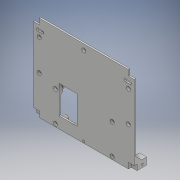
# Autodesk Inventor part: baseplate_jetson_core
Saved by Autodesk Inventor 2018 (Build 220112000, 112)
## iProperties
Created: 2018-05-14
Part Number: baseplate_jetson_core
Material: Generic
Document SubType Name: Modeling
Designer: bitbots
Density: 1 g/cm^3
Appearance: Default
Author: bitbots
Autodesk Inventor part; units mm, degrees
ref_plane "YZ Plane" through (0, 0, 0) normal (1, 0, 0) x (0, 1, 0)
ref_plane "XZ Plane" through (0, 0, 0) normal (0, 1, 0) x (-1, 0, 0)
ref_plane "XY Plane" through (0, 0, 0) normal (0, 0, 1) x (1, 0, 0)
sketch "Sketch1" plane through (0, 0, 0) normal (0, 1, 0) x (-1, 0, 0)
  line L0 (-70, 60) -> (70, 60)
  line L1 (70, 60) -> (70, -60)
  line L2 (70, -60) -> (-70, -60)
  line L3 (-70, -60) -> (-70, 60)
  line L4 (-70, 60) -> (70, -60) construction
  line L5 (70, 60) -> (-70, -60) construction
  point P0 (0, 0)
  dimension "d0" = 140
  dimension "d1" = 120
  constraints: 12 end point, 2 midpoint, 2 parallel, 1 horizontal, 1 perpendicular
  measures "d0" distance of L1.end L2.end
  measures "d1" distance of L0.end L1.end
extrude "Extrusion1" add sketch "Sketch1" along normal blind 2
sketch "Sketch2" plane through (0, 2, 0) normal (0, 1, 0) x (1, 0, 0)
  line L0 (0, 0) -> (0, 14) construction
  line L1 (0, 14) -> (39.5, 14) construction
  line L2 (39.5, 14) -> (-39.5, 14) construction
  line L3 (-39.5, 14) -> (-39.5, 56) construction
  line L4 (-39.5, 56) -> (39.5, 56) construction
  line L5 (39.5, 56) -> (39.5, 14) construction
  circle A0 centre (-39.5, 56) radius 1.75
  circle A1 centre (-39.5, 14) radius 1.75
  circle A2 centre (39.5, 14) radius 1.75
  circle A3 centre (39.5, 56) radius 1.75
  line L6 (70, 60) -> (-70, 60) projected
  dimension "d5" = 39.5
  dimension "d6" = 79
  dimension "d7" = 42
  dimension "d8" = 3.5
  dimension "d9" = 3.5
  dimension "d10" = 3.5
  dimension "d11" = 3.5
  dimension "d36" = 4
  constraints: 12 end point, 4 centre point, 4 coincident, 2 parallel, 2 perpendicular, 1 horizontal, 1 vertical
  measures "d5" distance of L0.end L1.end
  measures "d6" distance of L3.end L4.end
  measures "d7" distance of L2.end L3.end
  measures "d8" diameter of A0
  measures "d9" diameter of A1
  measures "d10" diameter of A2
  measures "d11" diameter of A3
  measures "d36" distance between parallel lines of L6 L4
extrude "Extrusion2" cut sketch "Sketch2" against normal through all
sketch "Sketch6" plane through (0, 2, 0) normal (0, 1, 0) x (1, 0, 0)
  circle A0 centre (39.5, 14) radius 1.75 projected
  circle A1 centre (-39.5, 56) radius 1.75 projected
  circle A2 centre (-39.5, 14) radius 1.75 projected
  circle A3 centre (39.5, 56) radius 1.75 projected
  line L0 (-70, -60) -> (70, -60) projected
  line L1 (70, -60) -> (70, 60) projected
  line L2 (70, 60) -> (-70, 60) projected
  line L3 (-70, 60) -> (-70, -60) projected
  line L4 (70, 60) -> (70, -60) projected
  line L5 (70, 60) -> (60, 60)
  line L6 (60, 60) -> (60, 50)
  line L7 (60, 50) -> (70, 50)
  line L8 (70, 50) -> (70, 60)
  point P0 (0, 0)
  dimension "d49" = 10
  dimension "d50" = 10
  constraints: 8 end point, 2 parallel, 1 horizontal, 1 perpendicular
  measures "d49" distance of L7.end L6.end
  measures "d50" distance of L6.end L5.end
extrude "Extrusion6" add sketch "Sketch6" along normal blind 15 contours L7 L6 L2 L1
sketch "Sketch8" plane through (70, 0, 60) normal (1, 0, 0) x (0, 0, -1)
  line L0 (120, 0) -> (0, 0) projected
  line L1 (120, 0) -> (120, 17) projected
  line L2 (110, 17) -> (120, 17) projected
  line L3 (110, 2) -> (110, 17) projected
  line L4 (0, 2) -> (110, 2) projected
  line L5 (0, 0) -> (0, 2) projected
  line L6 (110, 2) -> (110, 11)
  line L7 (110, 2) -> (110, 17) projected
  line L8 (110, 11) -> (116, 11)
  circle A0 centre (116, 11) radius 1.5
  point P0 (60, 0)
  dimension "d56" = 9
  dimension "d57" = 6
  dimension "d58" = 3
  constraints: 4 end point, 1 centre point, 1 coincident, 1 perpendicular, 1 point on line
  measures "d56" distance of L3.start L6.end
  measures "d57" distance of L6.end L8.end
  measures "d58" diameter of A0
extrude "Extrusion8" cut sketch "Sketch8" against normal blind 10 contours A0
mirror "Mirror1" about plane through (0, 0, 0) normal (1, 0, 0) of "Extrusion6", "Extrusion8"
chamfer "Chamfer1" distance 8 angle 45 4 edges at (-60, 2, -55) (60, 2, -55) (-65, 2, -50) (65, 2, -50)
sketch "Sketch9" plane through (0, 0, 0) normal (0, -1, 0) x (1, 0, 0)
  circle A0 centre (39.5, -14) radius 1.75 projected
  circle A1 centre (-39.5, -56) radius 1.75 projected
  circle A2 centre (-39.5, -14) radius 1.75 projected
  circle A3 centre (39.5, -56) radius 1.75 projected
  line L0 (70, 60) -> (-70, 60) projected
  line L1 (-70, 60) -> (-70, -60) projected
  line L2 (-70, -60) -> (70, -60) projected
  line L3 (70, -60) -> (70, 60) projected
  line L4 (-70, 60) -> (-70, -60) projected
  line L5 (-70, -60) -> (-62, -60)
  line L6 (-62, -60) -> (-62, -52)
  line L7 (-62, -52) -> (-70, -52)
  line L8 (-70, -52) -> (-70, -60)
  line L9 (70, -60) -> (60, -60) projected
  line L10 (70, -60) -> (60, -60)
  line L11 (70, -50) -> (70, -60)
  line L12 (70, 60) -> (62, 60)
  line L13 (62, 60) -> (62, 52)
  line L14 (62, 52) -> (70, 52)
  line L15 (70, 52) -> (70, 60)
  line L16 (70, 60) -> (-70, 60) projected
  line L17 (-70, 60) -> (-62, 60)
  line L18 (-62, 60) -> (-62, 52)
  line L19 (-62, 52) -> (-70, 52)
  line L20 (-70, 52) -> (-70, 60)
  line L21 (70, -60) -> (62, -60)
  line L22 (62, -60) -> (62, -52)
  line L23 (62, -52) -> (70, -52)
  line L24 (70, -52) -> (70, -60)
  point P0 (0, 0)
  dimension "d64" = 8
  dimension "d65" = 8
  dimension "d68" = 8
  dimension "d69" = 8
  dimension "d70" = 8
  dimension "d71" = 8
  dimension "d96" = 8
  dimension "d97" = 8
  constraints: 36 end point, 8 parallel, 5 horizontal, 4 perpendicular
  measures "d64" distance of L7.end L6.end
  measures "d65" distance of L6.end L5.end
  measures "d68" distance of L14.end L13.end
  measures "d69" distance of L13.end L12.end
  measures "d70" distance of L18.end L19.end
  measures "d71" distance of L17.end L18.end
  measures "d96" distance of L22.end L23.end
  measures "d97" distance of L21.end L22.end
extrude "Extrusion9" cut sketch "Sketch9" against normal blind 4 contours L3 L14 L13 L0 | L18 L19 L1 L0 | L3 L2 L22 L23 | L7 L6 L2 L1
sketch "Sketch10" plane through (0, 2, 0) normal (0, 1, 0) x (1, 0, 0)
  line L0 (-62, -60) -> (62, -60) projected
  line L1 (70, -52) -> (70, 42) projected
  line L2 (52, 42) -> (70, 42) projected
  line L3 (52, 60) -> (52, 42) projected
  line L4 (52, 60) -> (-52, 60) projected
  line L5 (-52, 42) -> (-52, 60) projected
  line L6 (-70, 42) -> (-52, 42) projected
  line L7 (-70, 42) -> (-70, -52) projected
  circle A0 centre (39.5, 14) radius 1.75 projected
  circle A1 centre (-39.5, 56) radius 1.75 projected
  circle A2 centre (-39.5, 14) radius 1.75 projected
  circle A3 centre (39.5, 56) radius 1.75 projected
  line L8 (-70, 60) -> (70, 60) projected
  line L9 (0, 60) -> (0, 57.5)
  circle A4 centre (0, 57.5) radius 1.5
  line L10 (62, -52) -> (70, -52) projected
  line L11 (-70, -52) -> (-62, -52) projected
  line L12 (-62, -52) -> (-62, -60) projected
  line L13 (62, -60) -> (62, -52) projected
  point P0 (0, 0)
  point P1 (-62, 60)
  point P2 (60, 60)
  dimension "d74" = 2.5
  dimension "d75" = 3
  constraints: 2 end point, 1 centre point, 1 coincident, 1 midpoint, 1 vertical
  measures "d74" distance of L9.start L9.end
  measures "d75" diameter of A4
extrude "Extrusion10" cut sketch "Sketch10" against normal blind 4 contours A4
sketch "Sketch13" plane through (0, 2, 0) normal (0, 1, 0) x (1, 0, 0)
  line L0 (-62, -60) -> (62, -60) projected
  line L1 (70, -52) -> (70, 42) projected
  line L2 (52, 42) -> (70, 42) projected
  line L3 (52, 60) -> (52, 42) projected
  line L4 (52, 60) -> (-52, 60) projected
  line L5 (-52, 42) -> (-52, 60) projected
  line L6 (-70, 42) -> (-52, 42) projected
  line L7 (-70, 42) -> (-70, -52) projected
  circle A0 centre (0, 57.5) radius 1.5 projected
  circle A1 centre (39.5, 14) radius 1.75 projected
  circle A2 centre (-39.5, 56) radius 1.75 projected
  circle A3 centre (-39.5, 14) radius 1.75 projected
  circle A4 centre (39.5, 56) radius 1.75 projected
  line L8 (-70, -60) -> (-61, -60)
  line L9 (-62, -60) -> (62, -60) projected
  line L10 (-61, -60) -> (-61, -45)
  line L11 (-64.5, -45) -> (-57.5, -45) construction
  line L12 (-64.5, -46.75) -> (-57.5, -46.75)
  line L13 (-57.5, -43.25) -> (-64.5, -43.25)
  arc A5 (-64.5, -43.25) -> (-64.5, -46.75) centre (-64.5, -45) ccw
  arc A6 (-57.5, -46.75) -> (-57.5, -43.25) centre (-57.5, -45) ccw
  line L14 (-70, -52) -> (-62, -52) projected
  line L15 (-62, -52) -> (-62, -60) projected
  line L16 (62, -60) -> (62, -52) projected
  line L17 (62, -52) -> (70, -52) projected
  point P0 (0, 0)
  dimension "d90" = 9
  dimension "d91" = 15
  dimension "d92" = 3.5
  dimension "d93" = 3.5
  constraints: 12 end point, 4 point on circle, 4 tangent, 2 centre point, 1 collinear, 1 horizontal, 1 midpoint, 1 parallel, 1 perpendicular
  measures "d90" distance of L8.start L8.end
  measures "d91" distance of L8.end L10.end
  measures "d92" distance of L10.end L11.end
  measures "d93" diameter of A6
extrude "Extrusion13" cut sketch "Sketch13" against normal blind 3 contours A5 L13 A6 L12
mirror "Mirror3" about plane through (0, 0, 0) normal (1, 0, 0) of "Extrusion13"
sketch "Sketch18" plane through (0, 2, 0) normal (0, 1, 0) x (1, 0, 0)
  circle A0 centre (0, 57.5) radius 1.5 projected
  circle A1 centre (39.5, 14) radius 1.75 projected
  circle A2 centre (-39.5, 56) radius 1.75 projected
  circle A3 centre (-39.5, 14) radius 1.75 projected
  circle A4 centre (39.5, 56) radius 1.75 projected
  arc A5 (-57.5, -46.75) -> (-57.5, -43.25) centre (-57.5, -45) ccw projected
  line L0 (-57.5, -46.75) -> (-64.5, -46.75) projected
  arc A6 (-64.5, -43.25) -> (-64.5, -46.75) centre (-64.5, -45) ccw projected
  line L1 (-64.5, -43.25) -> (-57.5, -43.25) projected
  arc A7 (57.5, -43.25) -> (57.5, -46.75) centre (57.5, -45) ccw projected
  line L2 (57.5, -43.25) -> (64.5, -43.25) projected
  arc A8 (64.5, -46.75) -> (64.5, -43.25) centre (64.5, -45) ccw projected
  line L3 (64.5, -46.75) -> (57.5, -46.75) projected
  line L4 (70, -52) -> (70, 42) projected
  line L5 (52, 42) -> (70, 42) projected
  line L6 (52, 60) -> (52, 42) projected
  line L7 (52, 60) -> (-52, 60) projected
  line L8 (-52, 42) -> (-52, 60) projected
  line L9 (-70, 42) -> (-52, 42) projected
  line L10 (-70, 42) -> (-70, -52) projected
  line L11 (-70, -52) -> (-62, -52) projected
  line L12 (-62, -52) -> (-62, -60) projected
  line L13 (-62, -60) -> (62, -60) projected
  line L14 (62, -60) -> (62, -52) projected
  line L15 (62, -52) -> (70, -52) projected
  circle A9 centre (39.5, 56) radius 1.75 projected
  line L16 (39.5, 56) -> (9.5, 56)
  line L17 (39.5, 56) -> (34.5, 56)
  line L18 (34.5, 56) -> (34.5, 26)
  line L19 (34.5, 56) -> (34.5, 65)
  line L20 (9.5, 56) -> (9.5, 26)
  line L21 (34.5, 65) -> (9.5, 65)
  line L22 (9.5, 65) -> (9.5, 26)
  line L23 (9.5, 26) -> (34.5, 26)
  line L24 (34.5, 26) -> (34.5, 65)
  circle A10 centre (-39.5, 14) radius 1.75 construction
  line L25 (-39.5, 14) -> (39.5, 56) construction
  circle A11 centre (39.5, 14) radius 1.75 construction
  circle A12 centre (-39.5, 56) radius 1.75 construction
  line L26 (39.5, 14) -> (-39.5, 56) construction
  line L27 (-9.5, 14) -> (-9.5, 44)
  line L28 (-34.5, 5) -> (-9.5, 5)
  line L29 (-9.5, 5) -> (-9.5, 44)
  line L30 (-9.5, 44) -> (-34.5, 44)
  line L31 (-34.5, 44) -> (-34.5, 5)
  point P0 (0, 0)
  point P1 (0, 35)
  dimension "d118" = 30
  dimension "d119" = 5
  dimension "d120" = 30
  dimension "d121" = 9
  constraints: 32 end point, 4 parallel, 3 vertical, 2 horizontal, 2 perpendicular, 1 midpoint, 1 point on line
  measures "d118" distance of L16.start L16.end
  measures "d119" distance of L16.start L17.end
  measures "d120" distance of L17.end L18.end
  measures "d121" distance of L17.end L19.end
extrude "Extrusion18" cut sketch "Sketch18" against normal blind 5 contours L29 L28 L31 L30 L27
sketch "Sketch21" plane through (0, 2, 0) normal (0, 1, 0) x (1, 0, 0)
  circle A0 centre (39.5, 14) radius 1.75 projected
  circle A1 centre (39.5, 56) radius 1.75 projected
  circle A2 centre (-39.5, 56) radius 1.75 projected
  circle A3 centre (-39.5, 14) radius 1.75 projected
  circle A4 centre (39.5, -2) radius 1.75 projected
  circle A5 centre (39.5, 56) radius 3.5
  circle A6 centre (-39.5, 14) radius 3.5
  circle A7 centre (-39.5, 56) radius 1.75 projected
  circle A8 centre (-39.5, 56) radius 3.5
  circle A9 centre (39.5, 14) radius 3.5
  point P0 (0, 0)
  dimension "d129" = 7
  dimension "d130" = 7
  dimension "d131" = 7
  dimension "d145" = 7
  constraints: 4 centre point, 4 coincident
  measures "d129" diameter of A5
  measures "d130" diameter of A6
  measures "d131" diameter of A8
  measures "d145" diameter of A9
extrude "Extrusion19" add sketch "Sketch21" along normal blind 13 contours A5 | A6 | A8 | A9
chamfer "Chamfer2" distance 5 angle 45 4 edges at (36, 2, -56) (-43, 2, -14) (-43, 2, -56) (36, 2, -14)
sketch "Sketch22" plane through (0, 0, 0) normal (0, -1, 0) x (1, 0, 0)
  circle A0 centre (39.5, -14) radius 1.75 projected
  circle A1 centre (-39.5, -14) radius 1.75 projected
  circle A2 centre (39.5, -14) radius 2.8
  circle A3 centre (-39.5, -14) radius 2.8
  line L0 (-9.5, -44) -> (-34.5, -44) construction
  line L1 (-34.5, -44) -> (-34.5, -5) construction
  line L2 (-34.5, -5) -> (-9.5, -5) construction
  line L3 (-9.5, -5) -> (-9.5, -44) construction
  arc A4 (57.5, 46.75) -> (57.5, 43.25) centre (57.5, 45) ccw construction
  line L4 (57.5, 46.75) -> (64.5, 46.75) construction
  arc A5 (64.5, 43.25) -> (64.5, 46.75) centre (64.5, 45) ccw construction
  line L5 (64.5, 43.25) -> (57.5, 43.25) construction
  arc A6 (-57.5, 43.25) -> (-57.5, 46.75) centre (-57.5, 45) ccw construction
  line L6 (-57.5, 43.25) -> (-64.5, 43.25) construction
  arc A7 (-64.5, 46.75) -> (-64.5, 43.25) centre (-64.5, 45) ccw construction
  line L7 (-64.5, 46.75) -> (-57.5, 46.75) construction
  circle A8 centre (0, -57.5) radius 1.5 construction
  line L8 (-62, -52) -> (-62, -60) construction
  line L9 (-62, -60) -> (62, -60) construction
  line L10 (62, -60) -> (62, -52) construction
  line L11 (62, -52) -> (70, -52) construction
  line L12 (70, -52) -> (70, 52) construction
  line L13 (70, 52) -> (62, 52) construction
  line L14 (62, 52) -> (62, 60) construction
  line L15 (62, 60) -> (-62, 60) construction
  line L16 (-62, 60) -> (-62, 52) construction
  line L17 (-62, 52) -> (-70, 52) construction
  line L18 (-70, 52) -> (-70, -52) construction
  line L19 (-70, -52) -> (-62, -52) construction
  circle A9 centre (39.5, -14) radius 1.75 construction
  circle A10 centre (-39.5, -56) radius 1.75 construction
  circle A11 centre (-39.5, -14) radius 1.75 construction
  circle A12 centre (39.5, -56) radius 1.75 construction
  circle A13 centre (39.5, -56) radius 1.75 projected
  circle A14 centre (39.5, -56) radius 2.8
  circle A15 centre (-39.5, -56) radius 2.8
  point P0 (0, 0)
  dimension "d137" = 5.6
  dimension "d138" = 5.6
  dimension "d172" = 5.6
  dimension "d173" = 5.6
  constraints: 4 centre point, 4 coincident
  measures "d137" diameter of A2
  measures "d138" diameter of A3
  measures "d172" diameter of A14
  measures "d173" diameter of A15
extrude "Extrusion20" cut sketch "Sketch22" against normal blind 3 contours A1 | A2 | A3 | A14 | A15
sketch "Sketch25" plane through (0, 2, 0) normal (0, 1, 0) x (1, 0, 0)
  circle A0 centre (39.5, 14) radius 8.5 construction
  arc A1 (-47, 60) -> (-32, 60) centre (-39.5, 56) ccw construction
  line L0 (-47, 60) -> (-52, 60) construction
  line L1 (-52, 42) -> (-52, 60) construction
  line L2 (-70, 42) -> (-52, 42) construction
  line L3 (-70, 42) -> (-70, -52) construction
  line L4 (-70, -52) -> (-62, -52) construction
  line L5 (-62, -52) -> (-62, -60) construction
  line L6 (-62, -60) -> (62, -60) construction
  line L7 (62, -60) -> (62, -52) construction
  line L8 (62, -52) -> (70, -52) construction
  line L9 (70, -52) -> (70, 42) construction
  line L10 (52, 42) -> (70, 42) construction
  line L11 (52, 60) -> (52, 42) construction
  line L12 (52, 60) -> (47, 60) construction
  arc A2 (32, 60) -> (47, 60) centre (39.5, 56) ccw construction
  line L13 (32, 60) -> (-32, 60) construction
  arc A3 (57.5, -43.25) -> (57.5, -46.75) centre (57.5, -45) ccw construction
  line L14 (57.5, -43.25) -> (64.5, -43.25) construction
  arc A4 (64.5, -46.75) -> (64.5, -43.25) centre (64.5, -45) ccw construction
  line L15 (64.5, -46.75) -> (57.5, -46.75) construction
  arc A5 (-57.5, -46.75) -> (-57.5, -43.25) centre (-57.5, -45) ccw construction
  line L16 (-57.5, -46.75) -> (-64.5, -46.75) construction
  arc A6 (-64.5, -43.25) -> (-64.5, -46.75) centre (-64.5, -45) ccw construction
  line L17 (-64.5, -43.25) -> (-57.5, -43.25) construction
  circle A7 centre (0, 57.5) radius 1.5 construction
  arc A8 (-34.5, 20.8739) -> (-34.5, 7.1261) centre (-39.5, 14) ccw construction
  line L18 (-34.5, 20.8739) -> (-34.5, 44) construction
  line L19 (-34.5, 44) -> (-9.5, 44) construction
  line L20 (-9.5, 44) -> (-9.5, 5) construction
  line L21 (-9.5, 5) -> (-34.5, 5) construction
  line L22 (-34.5, 5) -> (-34.5, 7.1261) construction
  line L23 (62, -52) -> (62, -37) construction
  line L24 (62, -37) -> (62, 6) construction
  line L25 (62, -37) -> (105, -37) construction
  circle A9 centre (62, 6) radius 1.6
  circle A10 centre (62, -37) radius 1.6
  line L26 (0, 0) -> (0, -80) construction
  line L27 (0, 0) -> (80, 0) construction
  circle A11 centre (-62, 6) radius 1.6
  circle A12 centre (-62, -37) radius 1.6
  line L28 (0, 0) -> (0, -52) construction
  circle A13 centre (0, -52) radius 1.6
  dimension "d146" = 15
  dimension "d148" = 43
  dimension "d149" = 90
  dimension "d150" = 3.2
  dimension "d151" = 3.2
  dimension "d152" = 80
  dimension "d153" = 90
  dimension "d154" = 52
  dimension "d155" = 3.2
  constraints: 12 end point, 5 centre point, 3 coincident, 3 vertical, 2 horizontal, 2 perpendicular, 2 symmetric about line, 1 point on line, 2 other
  measures "d146" distance of L7.end L23.end
  measures "d148" distance of L23.end L24.end
  measures "d149" angle of L25 L24
  measures "d150" diameter of A9
  measures "d151" diameter of A10
  measures "d152" distance of L26.start L26.end
  measures "d153" angle of L26 L27
  measures "d154" distance of L26.start L28.end
  measures "d155" diameter of A13
extrude "Extrusion22" cut sketch "Sketch25" against normal blind 10
sketch "Sketch26" plane through (0, 2, 0) normal (0, 1, 0) x (1, 0, 0)
  circle A0 centre (-62, 6) radius 1.6 projected
  circle A1 centre (62, -37) radius 1.6 construction
  circle A2 centre (62, 6) radius 1.6 construction
  circle A3 centre (-62, -37) radius 1.6 projected
  circle A4 centre (0, -52) radius 1.6 construction
  circle A5 centre (0, 57.5) radius 1.5 construction
  arc A6 (-57.5, -46.75) -> (-57.5, -43.25) centre (-57.5, -45) ccw construction
  line L0 (-57.5, -46.75) -> (-64.5, -46.75) construction
  arc A7 (-64.5, -43.25) -> (-64.5, -46.75) centre (-64.5, -45) ccw construction
  line L1 (-64.5, -43.25) -> (-57.5, -43.25) construction
  arc A8 (57.5, -43.25) -> (57.5, -46.75) centre (57.5, -45) ccw construction
  line L2 (57.5, -43.25) -> (64.5, -43.25) construction
  arc A9 (64.5, -46.75) -> (64.5, -43.25) centre (64.5, -45) ccw construction
  line L3 (64.5, -46.75) -> (57.5, -46.75) construction
  arc A10 (-34.5, 20.8739) -> (-34.5, 7.1261) centre (-39.5, 14) ccw construction
  line L4 (-34.5, 20.8739) -> (-34.5, 44) construction
  line L5 (-34.5, 44) -> (-9.5, 44) construction
  line L6 (-9.5, 44) -> (-9.5, 5) construction
  line L7 (-9.5, 5) -> (-34.5, 5) construction
  line L8 (-34.5, 5) -> (-34.5, 7.1261) construction
  arc A11 (-47, 60) -> (-32, 60) centre (-39.5, 56) ccw construction
  line L9 (-47, 60) -> (-52, 60) construction
  line L10 (-52, 42) -> (-52, 60) construction
  line L11 (-70, 42) -> (-52, 42) construction
  line L12 (-70, 42) -> (-70, -52) construction
  line L13 (-70, -52) -> (-62, -52) construction
  line L14 (-62, -52) -> (-62, -60) construction
  line L15 (-62, -60) -> (62, -60) construction
  line L16 (62, -60) -> (62, -52) construction
  line L17 (62, -52) -> (70, -52) construction
  line L18 (70, -52) -> (70, 42) construction
  line L19 (52, 42) -> (70, 42) construction
  line L20 (52, 60) -> (52, 42) construction
  line L21 (52, 60) -> (47, 60) construction
  arc A12 (32, 60) -> (47, 60) centre (39.5, 56) ccw construction
  line L22 (32, 60) -> (-32, 60) construction
  circle A13 centre (39.5, 14) radius 8.5 construction
  circle A14 centre (-62, -37) radius 1.6 construction
  circle A15 centre (-62, -37) radius 3.5
  circle A16 centre (-62, 6) radius 3.5
  circle A17 centre (62, -37) radius 1.6 projected
  circle A18 centre (62, -37) radius 3.5
  circle A19 centre (62, 6) radius 1.6 projected
  circle A20 centre (62, 6) radius 3.5
  circle A21 centre (0, -52) radius 1.6 projected
  circle A22 centre (0, -52) radius 3.5
  point P0 (0, 0)
  dimension "d158" = 7
  dimension "d159" = 7
  dimension "d160" = 7
  dimension "d161" = 7
  dimension "d162" = 7
  constraints: 5 centre point, 5 coincident
  measures "d158" diameter of A15
  measures "d159" diameter of A16
  measures "d160" diameter of A18
  measures "d161" diameter of A20
  measures "d162" diameter of A22
extrude "Extrusion23" add sketch "Sketch26" along normal blind 4
sketch "Sketch27" plane through (0, 0, 0) normal (0, -1, 0) x (1, 0, 0)
  circle A0 centre (-62, -6) radius 1.6 construction
  circle A1 centre (62, 37) radius 1.6 construction
  circle A2 centre (62, -6) radius 1.6 construction
  circle A3 centre (-62, 37) radius 1.6 construction
  circle A4 centre (0, 52) radius 1.6 construction
  circle A5 centre (-39.5, -14) radius 2.8 construction
  circle A6 centre (39.5, -14) radius 2.8 construction
  line L0 (-9.5, -44) -> (-34.5, -44) construction
  line L1 (-34.5, -44) -> (-34.5, -5) construction
  line L2 (-34.5, -5) -> (-9.5, -5) construction
  line L3 (-9.5, -5) -> (-9.5, -44) construction
  arc A7 (57.5, 46.75) -> (57.5, 43.25) centre (57.5, 45) ccw construction
  line L4 (57.5, 46.75) -> (64.5, 46.75) construction
  arc A8 (64.5, 43.25) -> (64.5, 46.75) centre (64.5, 45) ccw construction
  line L5 (64.5, 43.25) -> (57.5, 43.25) construction
  arc A9 (-57.5, 43.25) -> (-57.5, 46.75) centre (-57.5, 45) ccw construction
  line L6 (-57.5, 43.25) -> (-64.5, 43.25) construction
  arc A10 (-64.5, 46.75) -> (-64.5, 43.25) centre (-64.5, 45) ccw construction
  line L7 (-64.5, 46.75) -> (-57.5, 46.75) construction
  circle A11 centre (0, -57.5) radius 1.5 construction
  line L8 (-62, -52) -> (-62, -60) construction
  line L9 (-62, -60) -> (62, -60) construction
  line L10 (62, -60) -> (62, -52) construction
  line L11 (62, -52) -> (70, -52) construction
  line L12 (70, -52) -> (70, 52) construction
  line L13 (70, 52) -> (62, 52) construction
  line L14 (62, 52) -> (62, 60) construction
  line L15 (62, 60) -> (-62, 60) construction
  line L16 (-62, 60) -> (-62, 52) construction
  line L17 (-62, 52) -> (-70, 52) construction
  line L18 (-70, 52) -> (-70, -52) construction
  line L19 (-70, -52) -> (-62, -52) construction
  circle A12 centre (62, 37) radius 1.6 construction
  circle A13 centre (62, 37) radius 2.8
  circle A14 centre (62, -6) radius 2.8
  circle A15 centre (0, 52) radius 1.6 projected
  circle A16 centre (0, 52) radius 2.8
  circle A17 centre (-62, 37) radius 1.6 projected
  circle A18 centre (-62, 37) radius 2.8
  circle A19 centre (-62, -6) radius 1.6 projected
  circle A20 centre (-62, -6) radius 2.8
  point P0 (0, 0)
  dimension "d165" = 5.6
  dimension "d166" = 5.6
  dimension "d167" = 5.6
  dimension "d168" = 5.6
  dimension "d169" = 5.6
  constraints: 5 centre point, 5 coincident
  measures "d165" diameter of A13
  measures "d166" diameter of A14
  measures "d167" diameter of A16
  measures "d168" diameter of A18
  measures "d169" diameter of A20
extrude "Extrusion24" cut sketch "Sketch27" against normal blind 3
body "Solid1"
